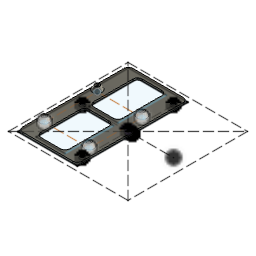
pi sled (Autodesk Fusion 360 design; units mm, degrees)
Autodesk Fusion 360 part; units mm, degrees
sketch "Sketch1" plane through (0, 0, 0) normal (0, 0, 1) x (1, 0, 0)
  line L0 (65.5, -65.5) -> (-65.5, -65.5) construction
  line L1 (-65.5, -65.5) -> (-65.5, 65.5) construction
  line L2 (-65.5, 65.5) -> (65.5, 65.5) construction
  line L3 (65.5, 65.5) -> (65.5, -65.5) construction
  line L4 (65.5, -65.5) -> (-65.5, 65.5) construction
  line L5 (-65.5, -65.5) -> (65.5, 65.5) construction
  line L6 (0, 50) -> (0, -50) construction
  line L7 (-50, 0) -> (50, 0) construction
  line L8 (-60, 60.5) -> (5, 60.5)
  line L9 (5, 60.5) -> (5, -60.5)
  line L10 (5, -60.5) -> (-60, -60.5)
  line L11 (-60, -60.5) -> (-60, 60.5)
  circle A0 centre (-50, 0) radius 2.5
  circle A1 centre (0, 50) radius 2.5
  circle A2 centre (0, -50) radius 2.5
  line L12 (-54.4646, 20.8308) -> (-5.4646, 20.8308) construction
  line L13 (-5.4646, 20.8308) -> (-5.4646, -37.1692) construction
  line L14 (-5.4646, -37.1692) -> (-54.4646, -37.1692) construction
  line L15 (-54.4646, -37.1692) -> (-54.4646, 20.8308) construction
  circle A3 centre (-54.4646, 20.8308) radius 1.15
  circle A4 centre (-54.4646, 20.8308) radius 2.65
  circle A5 centre (-5.4646, 20.8308) radius 1.15
  circle A6 centre (-5.4646, 20.8308) radius 2.65
  circle A7 centre (-54.4646, -37.1692) radius 1.15
  circle A8 centre (-54.4646, -37.1692) radius 2.65
  circle A9 centre (-5.4646, -37.1692) radius 1.15
  circle A10 centre (-5.4646, -37.1692) radius 2.65
  line L16 (-45, 2.5) -> (-13.4646, 2.5)
  line L17 (-13.4646, 2.5) -> (-13.4646, 55.5)
  line L18 (-13.4646, 55.5) -> (-45, 55.5)
  line L19 (-45, 55.5) -> (-45, 2.5)
  line L20 (-45, -2.5) -> (-13.4646, -2.5)
  line L21 (-13.4646, -2.5) -> (-13.4646, -55.5)
  line L22 (-13.4646, -55.5) -> (-45, -55.5)
  line L23 (-45, -55.5) -> (-45, -2.5)
  point P0 (5, 0)
  dimension "d4" = 131
  dimension "d5" = 131
  dimension "d6" = 100
  dimension "d7" = 100
  dimension "d8" = 5
  dimension "d9" = 5
  dimension "d10" = 5
  dimension "d14" = 5
  dimension "d15" = 10
  dimension "d16" = 49
  dimension "d17" = 58
  dimension "d18" = 2.3
  dimension "d19" = 1.5
  dimension "d22" = 49
  dimension "d23" = -58
  dimension "d32" = 5
  dimension "d33" = 5
  dimension "d35" = 8
  dimension "d36" = 2.5
  dimension "d37" = 2.5
  dimension "d38" = 5
  dimension "d39" = 5
  dimension "d40" = 8
  dimension "d41" = 5
  dimension "d42" = 5
  constraint horizontal L0
  constraint perpendicular L0 L1
  constraint parallel L0 L2
  constraint parallel L1 L3
  constraint coincident L4 origin
  constraint coincident L5 origin
  constraint vertical L6
  constraint horizontal L7
  constraint midpoint origin L7
  constraint midpoint origin L6
  constraint horizontal L8
  constraint vertical L9
  constraint horizontal L10
  constraint vertical L11
  constraint coincident L7.start A0.centre
  constraint coincident L6.start A1.centre
  constraint coincident L6.end A2.centre
  constraint midpoint L9 P0
  constraint coincident L7 P0
  constraint horizontal L12
  constraint vertical L13
  constraint horizontal L14
  constraint vertical L15
  constraint coincident L12.start L15.end
  constraint horizontal L16
  constraint vertical L17
  constraint horizontal L18
  constraint vertical L19
  constraint horizontal L20
  constraint vertical L21
  constraint horizontal L22
  constraint vertical L23
  measures "d4" distance of L1.end L2.end
  measures "d5" distance of L0.end L1.end
  measures "d6" distance of L6.start L6.end
  measures "d7" distance of L7.start L7.end
  measures "d8" diameter of A0
  measures "d9" diameter of A1
  measures "d10" diameter of A2
  measures "d14" distance of L9 L6.end
  measures "d15" distance of L11 L7.start
  measures "d16" distance of L12.start L12.end
  measures "d17" distance of L12.start L14.end
  measures "d18" diameter of A3
  measures "d19" distance of A3 A4
  measures "d32" distance of L7.start L19
  measures "d33" distance of L8 L18
  measures "d35" distance of L12.end L17
  measures "d36" distance of L7 L16
  measures "d37" distance of L7 L20
  measures "d38" distance of L10 L22
  measures "d39" distance of L7.start L23
  measures "d40" distance of L12.end L21
  measures "d41" distance of L2 L8
  measures "d42" distance of L0 L10
extrude "Extrude1" add sketch "Sketch1" along normal blind 2 contours L8 L9 L10 L11 | A3 | A4 | A5 | A6 | A7 | A8 | A9 | A10
extrude "Extrude2" add sketch "Sketch1" along normal blind 6.5 contours A4 | A6 | A8 | A10
draft "Draft1" angle 30 neutral plane through (0, 0, 6.5) pull (0, 0, 1) 4 faces at (-51.8278, -36.9053, 3.5) (-51.8278, 21.0947, 3.5) (-2.8278, 21.0947, 3.5) (-2.8278, -36.9053, 3.5)
fillet "Fillet1" radius 5 12 edges at (-60, -60.5, 1) (5, -60.5, 1) (5, 60.5, 1) (-60, 60.5, 1) (-45, 55.5, 1) (-13.4646, 55.5, 1) (-13.4646, 2.5, 1) (-45, 2.5, 1) (-45, -2.5, 1) (-13.4646, -2.5, 1) (-13.4646, -55.5, 1) (-45, -55.5, 1)
